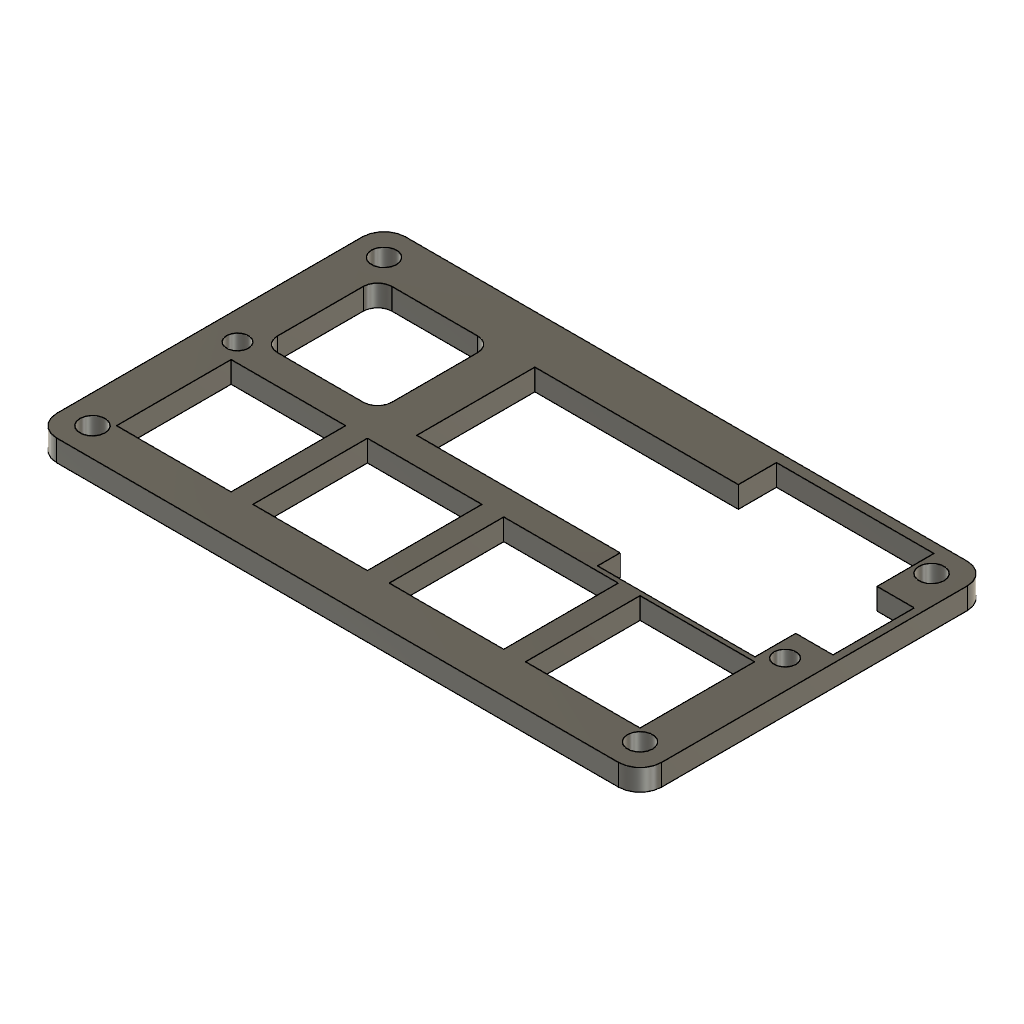
Hayai full bulid V1 (Autodesk Fusion 360 archive; units mm, degrees)
design "Hayai Upper midplate"
part number: 2026-09-20-16-56-58-125
Autodesk Fusion 360 part; units mm, degrees
note: some values were not read from the file. Chosen so that the rebuilt part matches the saved one: which face or edge a step refers to. Set by a fixed rule: which sketch regions a step uses.
(part 1 of 2)
sketch "Sketch1" plane through (0, 0, 0) normal (0, 0, 1) x (1, 0, 0)
  circle A0 centre (-38.26, 20.3675) radius 1.75
  circle A1 centre (38.26, 20.3675) radius 1.75
  circle A2 centre (38.26, -20.3675) radius 1.75
  circle A3 centre (-38.26, -20.3675) radius 1.75
  line L0 (14, 22.9575) -> (36, 22.9575)
  line L1 (36, 15) -> (36, 22.9575)
  line L2 (36, 15) -> (41.21, 15)
  line L3 (41.21, 15) -> (41.21, 3.65)
  line L4 (41.21, 3.65) -> (36, 3.65)
  line L5 (36, -2.0425) -> (36, 3.65)
  line L6 (36, -2.0425) -> (14, -2.0425)
  line L7 (-14.435, 1.1275) -> (-14.435, 17.6275)
  line L8 (-14.435, 1.1275) -> (14, 1.1275)
  line L9 (-14.435, 17.6275) -> (14, 17.6275)
  line L10 (14, -2.0425) -> (14, 1.1275)
  line L11 (14, 17.6275) -> (14, 22.9575)
  circle A4 centre (-38.26, -0.0995) radius 1.525
  circle A5 centre (38.26, -0.0995) radius 1.525
  line L12 (-39.26, 24.3675) -> (39.26, 24.3675)
  line L13 (42.26, 21.3675) -> (42.26, -21.3675)
  line L14 (39.26, -24.3675) -> (-39.26, -24.3675)
  line L15 (-42.26, -21.3675) -> (-42.26, 21.3675)
  arc A6 (-39.26, 24.3675) -> (-42.26, 21.3675) centre (-39.26, 21.3675) ccw
  arc A7 (42.26, 21.3675) -> (39.26, 24.3675) centre (39.26, 21.3675) ccw
  arc A8 (39.26, -24.3675) -> (42.26, -21.3675) centre (39.26, -21.3675) ccw
  arc A9 (-42.26, -21.3675) -> (-39.26, -24.3675) centre (-39.26, -21.3675) ccw
  line L16 (-22.19, 1.4035) -> (-34.19, 1.4035)
  line L17 (-36.19, 3.4035) -> (-36.19, 15.4035)
  line L18 (-34.19, 17.4035) -> (-22.19, 17.4035)
  line L19 (-20.19, 15.4035) -> (-20.19, 3.4035)
  line L20 (-20.19, 1.4035) -> (-36.19, 17.4035) construction
  line L21 (-36.19, 1.4035) -> (-20.19, 17.4035) construction
  arc A10 (-34.19, 17.4035) -> (-36.19, 15.4035) centre (-34.19, 15.4035) ccw
  arc A11 (-22.19, 1.4035) -> (-20.19, 3.4035) centre (-22.19, 3.4035) ccw
  arc A12 (-36.19, 3.4035) -> (-34.19, 1.4035) centre (-34.19, 3.4035) ccw
  arc A13 (-20.19, 15.4035) -> (-22.19, 17.4035) centre (-22.19, 15.4035) ccw
  line L22 (20.575, -18.6825) -> (36.575, -18.6825)
  line L23 (36.575, -18.6825) -> (36.575, -2.6825)
  line L24 (36.575, -2.6825) -> (20.575, -2.6825)
  line L25 (20.575, -2.6825) -> (20.575, -18.6825)
  line L26 (20.575, -18.6825) -> (36.575, -2.6825) construction
  line L27 (36.575, -18.6825) -> (20.575, -2.6825) construction
  line L28 (1.525, -18.6825) -> (17.525, -18.6825)
  line L29 (17.525, -18.6825) -> (17.525, -2.6825)
  line L30 (17.525, -2.6825) -> (1.525, -2.6825)
  line L31 (1.525, -2.6825) -> (1.525, -18.6825)
  line L32 (1.525, -18.6825) -> (17.525, -2.6825) construction
  line L33 (17.525, -18.6825) -> (1.525, -2.6825) construction
  line L34 (-17.525, -18.6825) -> (-1.525, -18.6825)
  line L35 (-1.525, -18.6825) -> (-1.525, -2.6825)
  line L36 (-1.525, -2.6825) -> (-17.525, -2.6825)
  line L37 (-17.525, -2.6825) -> (-17.525, -18.6825)
  line L38 (-17.525, -18.6825) -> (-1.525, -2.6825) construction
  line L39 (-1.525, -18.6825) -> (-17.525, -2.6825) construction
  line L40 (-36.575, -18.6825) -> (-20.575, -18.6825)
  line L41 (-20.575, -18.6825) -> (-20.575, -2.6825)
  line L42 (-20.575, -2.6825) -> (-36.575, -2.6825)
  line L43 (-36.575, -2.6825) -> (-36.575, -18.6825)
  line L44 (-36.575, -18.6825) -> (-20.575, -2.6825) construction
  line L45 (-20.575, -18.6825) -> (-36.575, -2.6825) construction
  point P0 (1.0651, 9.3775)
  point P1 (-28.19, 9.4035)
  point P2 (-28.19, 9.4035)
  point P3 (42.26, -24.3675)
  point P4 (-42.26, 24.3675)
  point P5 (-28.19, 9.4035)
  point P6 (-28.19, 9.4035)
  point P7 (28.575, -10.6825)
  point P8 (9.525, -10.6825)
  point P9 (-28.575, -10.6825)
  point P10 (-9.525, -10.6825)
  point P11 (28.575, -10.6825)
  point P12 (9.525, -10.6825)
  point P13 (-9.525, -10.6825)
  point P14 (-28.575, -10.6825)
  dimension "d2" = 3.5
  dimension "d11" = 22
  dimension "d12" = 25
  dimension "d13" = 5.21
  dimension "d14" = 11.35
  dimension "d18" = 16.5
  dimension "d31" = 3.05
  dimension "d32" = 3.05
  dimension "d33" = 20.268
  dimension "d34" = 20.268
  dimension "d53" = 3
  dimension "d54" = 3
  dimension "d55" = 3
  dimension "d56" = 3
  dimension "d67" = 84.52
  dimension "d68" = 14.07
  dimension "d69" = 14.964
  dimension "d70" = 16
  dimension "d71" = 16
  dimension "d72" = 2
  dimension "d73" = 2
  dimension "d74" = 2
  dimension "d75" = 2
  dimension "d80" = 19.05
  dimension "d81" = 16
  dimension "d82" = 16
  dimension "d83" = 16
  dimension "d84" = 16
  dimension "d85" = 16
  dimension "d86" = 16
  dimension "d87" = 16
  dimension "d88" = 16
  constraint horizontal L0
  constraint horizontal L6
  constraint horizontal L2
  constraint vertical L3
  constraint horizontal L4
  constraint perpendicular L8 L10
  constraint coincident P6 P5
  constraint horizontal L12
  constraint vertical L13
  constraint horizontal L14
  constraint vertical L15
  constraint tangent L12 A6
  constraint tangent L15 A6
  constraint tangent L12 A7
  constraint tangent L13 A7
  constraint tangent L13 A8
  constraint tangent L14 A8
  constraint tangent L14 A9
  constraint tangent L15 A9
  constraint horizontal L16
  constraint perpendicular L16 L17
  constraint parallel L16 L18
  constraint parallel L17 L19
  constraint coincident L20 P6
  constraint coincident L21 P6
  constraint coincident L20.end L18
  constraint coincident L20.end L17
  constraint tangent L18 A10
  constraint tangent L17 A10
  constraint coincident L20.start L16
  constraint coincident L20.start L19
  constraint tangent L16 A11
  constraint tangent L19 A11
  constraint coincident L21.start L16
  constraint coincident L21.start L17
  constraint tangent L16 A12
  constraint tangent L17 A12
  constraint coincident L21.end L18
  constraint coincident L21.end L19
  constraint tangent L18 A13
  constraint tangent L19 A13
  constraint horizontal L22
  constraint perpendicular L22 L23
  constraint parallel L22 L24
  constraint parallel L23 L25
  constraint coincident L26 P11
  constraint coincident L27 P11
  constraint coincident P11 P7
  constraint horizontal L28
  constraint perpendicular L28 L29
  constraint parallel L28 L30
  constraint parallel L29 L31
  constraint coincident L32 P12
  constraint coincident L33 P12
  constraint coincident P12 P8
  constraint horizontal L34
  constraint perpendicular L34 L35
  constraint parallel L34 L36
  constraint parallel L35 L37
  constraint coincident L38 P13
  constraint coincident L39 P13
  constraint coincident P13 P10
  constraint horizontal L40
  constraint perpendicular L40 L41
  constraint parallel L40 L42
  constraint parallel L41 L43
  constraint coincident L44 P14
  constraint coincident L45 P14
  constraint coincident P14 P9
  constraint equal A0 A3
  constraint equal A0 A2
  constraint equal A0 A1
  measures "d2" diameter of A0
  measures "d11" distance of L0.end L0.start
  measures "d12" distance of L6.end L0.start
  measures "d13" distance of L1.start L2.end
  measures "d14" distance of L1.start L4.end
  measures "d18" distance of L7.start L7.end
  measures "d31" diameter of A4
  measures "d32" diameter of A5
  measures "d33" distance of A2.centre A5.centre
  measures "d34" distance of A3.centre A4.centre
  measures "d53" radius of A6
  measures "d54" radius of A7
  measures "d55" radius of A8
  measures "d56" radius of A9
  measures "d67" distance of L13 L15
  measures "d68" distance of L15 P6
  measures "d69" distance of L12 P6
  measures "d70" distance of L20.end L21.end
  measures "d71" distance of L21.start L20.end
  measures "d72" radius of A10
  measures "d73" radius of A11
  measures "d74" radius of A12
  measures "d75" radius of A13
  measures "d80" distance of P14 P13
  measures "d81" distance of L23.end L24.end
  measures "d82" distance of L22.end L23.end
  measures "d83" distance of L29.end L30.end
  measures "d84" distance of L28.end L29.end
  measures "d85" distance of L35.end L36.end
  measures "d86" distance of L34.end L35.end
  measures "d87" distance of L41.end L42.end
  measures "d88" distance of L40.end L41.end
extrude "Extrude13" add sketch "Sketch1" along normal blind 3 contours L12 L13 L14 L15 A6 A7 A8 A9 | L16 L17 L18 L19 A10 A11 A12 A13 | L22 L23 L24 L25 | L28 L29 L30 L31 | L34 L35 L36 L37 | L40 L41 L42 L43 makes body 1
extrude "Extrude14" add sketch "Sketch1" along normal blind 3 separate body contours L12 L13 L14 L15 A6 A7 A8 A9 | L22 L23 L24 L25 | L28 L29 L30 L31 | L34 L35 L36 L37 | L40 L41 L42 L43 makes body 2
extrude "Extrude15" cut sketch "Sketch1" along normal blind 3 contours L16 L17 L18 L19 A10 A11 A12 A13 bodies 1
extrude "Extrude16" add sketch "Sketch1" along normal blind 3 separate body makes body 3
extrude "Extrude17" cut sketch "Sketch1" along normal blind 3 contours L22 L23 L24 L25 | L28 L29 L30 L31 | L34 L35 L36 L37 | L40 L41 L42 L43 bodies 1 2
extrude "Extrude18" add sketch "Sketch1" along normal blind 3 separate body makes body 4

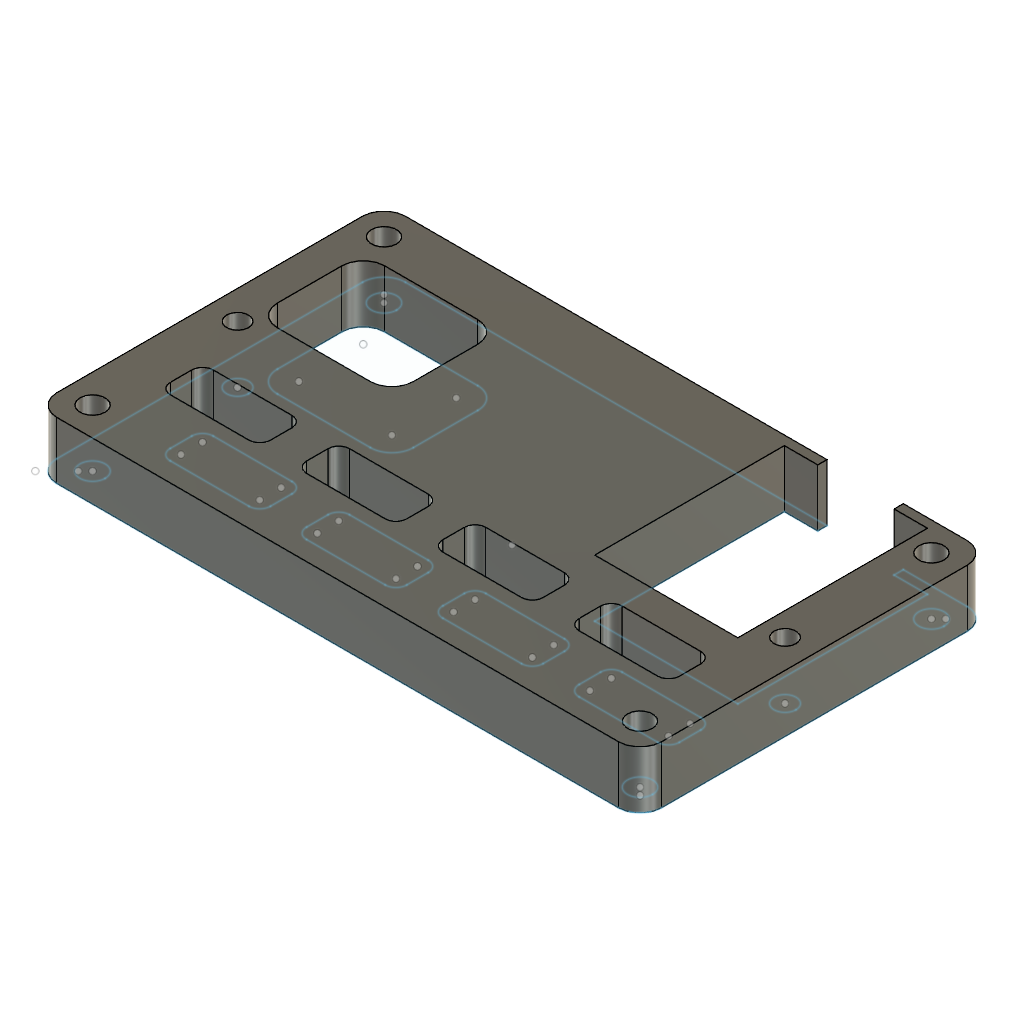
design "Hayai Lower midplate"
part number: 2026-09-20-19-27-11-121
Autodesk Fusion 360 part; units mm, degrees
sketch "Sketch1" plane through (0, 0, 0) normal (0, 0, 1) x (1, 0, 0)
  arc A0 (39.26, -24.3675) -> (42.26, -21.3675) centre (39.26, -21.3675) ccw
  circle A1 centre (38.26, -0.0995) radius 1.525
  circle A2 centre (-38.26, -20.3675) radius 1.75
  circle A3 centre (-38.26, 20.3675) radius 1.75
  line L0 (42.26, 21.3675) -> (42.26, -21.3675)
  arc A4 (-42.26, -21.3675) -> (-39.26, -24.3675) centre (-39.26, -21.3675) ccw
  line L1 (39.26, -24.3675) -> (-39.26, -24.3675)
  line L2 (-42.26, -21.3675) -> (-42.26, 21.3675)
  arc A5 (-39.26, 24.3675) -> (-42.26, 21.3675) centre (-39.26, 21.3675) ccw
  arc A6 (42.26, 21.3675) -> (39.26, 24.3675) centre (39.26, 21.3675) ccw
  circle A7 centre (38.26, 20.3675) radius 1.75
  circle A8 centre (-38.26, -0.0995) radius 1.525
  circle A9 centre (38.26, -20.3675) radius 1.75
  arc A10 (16.525, -9.1875) -> (15.025, -7.6875) centre (15.025, -9.1875) ccw
  arc A11 (-35.575, -12.1875) -> (-34.075, -13.6875) centre (-34.075, -12.1875) ccw
  line L3 (4.025, -7.6875) -> (15.025, -7.6875)
  arc A12 (-15.025, -7.6875) -> (-16.525, -9.1875) centre (-15.025, -9.1875) ccw
  line L4 (-16.525, -12.1875) -> (-16.525, -9.1875)
  line L5 (23.075, -13.6875) -> (34.075, -13.6875)
  line L6 (-15.025, -13.6875) -> (-4.025, -13.6875)
  arc A13 (21.575, -12.1875) -> (23.075, -13.6875) centre (23.075, -12.1875) ccw
  line L7 (-34.075, -7.6875) -> (-23.075, -7.6875)
  arc A14 (34.075, -13.6875) -> (35.575, -12.1875) centre (34.075, -12.1875) ccw
  line L8 (-34.075, -13.6875) -> (-23.075, -13.6875)
  line L9 (2.525, -12.1875) -> (2.525, -9.1875)
  arc A15 (35.575, -9.1875) -> (34.075, -7.6875) centre (34.075, -9.1875) ccw
  arc A16 (-2.525, -9.1875) -> (-4.025, -7.6875) centre (-4.025, -9.1875) ccw
  arc A17 (4.025, -7.6875) -> (2.525, -9.1875) centre (4.025, -9.1875) ccw
  line L10 (-35.575, -12.1875) -> (-35.575, -9.1875)
  line L11 (16.525, -12.1875) -> (16.525, -9.1875)
  arc A18 (-4.025, -13.6875) -> (-2.525, -12.1875) centre (-4.025, -12.1875) ccw
  line L12 (23.075, -7.6875) -> (34.075, -7.6875)
  arc A19 (-23.075, -13.6875) -> (-21.575, -12.1875) centre (-23.075, -12.1875) ccw
  line L13 (21.575, -12.1875) -> (21.575, -9.1875)
  line L14 (-15.025, -7.6875) -> (-4.025, -7.6875)
  line L15 (35.575, -12.1875) -> (35.575, -9.1875)
  arc A20 (2.525, -12.1875) -> (4.025, -13.6875) centre (4.025, -12.1875) ccw
  arc A21 (-16.525, -12.1875) -> (-15.025, -13.6875) centre (-15.025, -12.1875) ccw
  arc A22 (-21.575, -9.1875) -> (-23.075, -7.6875) centre (-23.075, -9.1875) ccw
  line L16 (-21.575, -12.1875) -> (-21.575, -9.1875)
  line L17 (-2.525, -12.1875) -> (-2.525, -9.1875)
  arc A23 (15.025, -13.6875) -> (16.525, -12.1875) centre (15.025, -12.1875) ccw
  arc A24 (-34.075, -7.6875) -> (-35.575, -9.1875) centre (-34.075, -9.1875) ccw
  line L18 (4.025, -13.6875) -> (15.025, -13.6875)
  arc A25 (23.075, -7.6875) -> (21.575, -9.1875) centre (23.075, -9.1875) ccw
  line L19 (-18.69, 4.8975) -> (-18.69, 13.8975)
  arc A26 (-18.69, 13.8975) -> (-21.69, 16.8975) centre (-21.69, 13.8975) ccw
  line L20 (-21.69, 16.8975) -> (-34.69, 16.8975)
  arc A27 (-34.69, 16.8975) -> (-37.69, 13.8975) centre (-34.69, 13.8975) ccw
  line L21 (-37.69, 4.8975) -> (-37.69, 13.8975)
  arc A28 (-37.69, 4.8975) -> (-34.69, 1.8975) centre (-34.69, 4.8975) ccw
  line L22 (-21.69, 1.8975) -> (-34.69, 1.8975)
  arc A29 (-21.69, 1.8975) -> (-18.69, 4.8975) centre (-21.69, 4.8975) ccw
  line L23 (35, -3.4325) -> (15, -3.4325)
  line L24 (19.67, 23.0675) -> (15, 23.0675)
  line L25 (30.33, 23.0675) -> (35, 23.0675)
  line L26 (15, -3.4325) -> (15, 23.0675)
  line L27 (35, 23.0675) -> (35, -3.4325)
  line L28 (19.67, 23.0675) -> (19.67, 24.3675)
  line L29 (30.33, 23.0675) -> (30.33, 24.3675)
  line L30 (39.26, 24.3675) -> (30.33, 24.3675)
  line L31 (19.67, 24.3675) -> (-39.26, 24.3675)
  point P0 (-42.26, -24.3675)
  dimension "d1" = 3.5
  dimension "d2" = 3.05
  dimension "d3" = 3.05
  dimension "d4" = 20.268
  dimension "d5" = 3
  dimension "d6" = 3
  dimension "d7" = 3
  dimension "d8" = 3
  dimension "d11" = 3.5
  dimension "d12" = 1.4142
  dimension "d13" = 4
  dimension "d14" = 10.68
  dimension "d15" = 6
  dimension "d16" = 14
  dimension "d17" = 1.5
  dimension "d18" = 1.5
  dimension "d19" = 1.5
  dimension "d20" = 1.5
  dimension "d21" = 1.5
  dimension "d22" = 1.5
  dimension "d23" = 1.5
  dimension "d24" = 1.5
  dimension "d25" = 1.5
  dimension "d26" = 1.5
  dimension "d27" = 1.5
  dimension "d28" = 1.5
  dimension "d29" = 1.5
  dimension "d30" = 1.5
  dimension "d31" = 1.5
  dimension "d32" = 1.5
  dimension "d33" = 6
  dimension "d34" = 6
  dimension "d35" = 6
  dimension "d36" = 10.68
  dimension "d37" = 10.68
  dimension "d38" = 10.68
  dimension "d40" = 6.685
  dimension "d41" = 5.05
  dimension "d42" = 5.05
  dimension "d43" = 5.05
  dimension "d44" = 4
  dimension "d45" = 4
  dimension "d46" = 4
  dimension "d47" = 1.4142
  dimension "d48" = 4
  dimension "d49" = 1.4142
  dimension "d50" = 20.268
  dimension "d51" = 14
  dimension "d52" = 14
  dimension "d53" = 14
  dimension "d54" = 6.685
  dimension "d55" = 3
  dimension "d56" = 3
  dimension "d57" = 3
  dimension "d58" = 3
  dimension "d59" = 19
  dimension "d60" = 15
  dimension "d61" = 4.57
  dimension "d63" = 26.5
  dimension "d64" = 26.5
  dimension "d65" = 20
  dimension "d66" = 10.66
  dimension "d67" = 1.3
  dimension "d68" = 1.3
  dimension "d69" = 4.67
  dimension "d70" = 4.67
  dimension "d71" = 7.26
  dimension "d78" = 3.5
  dimension "d79" = 3.5
  constraint vertical L0
  constraint horizontal L1
  constraint vertical L2
  constraint tangent L2 A5
  constraint tangent L0 A6
  constraint tangent A0 L0
  constraint tangent A0 L1
  constraint tangent A4 L1
  constraint tangent A4 L2
  constraint tangent A6 L30
  constraint tangent A5 L31
  measures "d1" diameter of A3
  measures "d2" diameter of A8
  measures "d3" diameter of A1
  measures "d4" distance of A2.centre A8.centre
  measures "d5" radius of A5
  measures "d6" radius of A6
  measures "d7" radius of A0
  measures "d8" radius of A4
  measures "d11" diameter of A9
  measures "d12" distance of A0.centre A9.centre
  measures "d13" distance of L1 A9.centre
  measures "d14" distance of L1 L8
  measures "d15" distance of L7 L8
  measures "d16" distance of L10 L16
  measures "d17" radius of A19
  measures "d18" radius of A22
  measures "d19" radius of A24
  measures "d20" radius of A11
  measures "d21" radius of A21
  measures "d22" radius of A12
  measures "d23" radius of A16
  measures "d24" radius of A18
  measures "d25" radius of A20
  measures "d26" radius of A17
  measures "d27" radius of A10
  measures "d28" radius of A23
  measures "d29" radius of A13
  measures "d30" radius of A25
  measures "d31" radius of A15
  measures "d32" radius of A14
  measures "d33" distance of L6 L14
  measures "d34" distance of L3 L18
  measures "d35" distance of L5 L12
  measures "d36" distance of L1 L6
  measures "d37" distance of L1 L5
  measures "d38" distance of L1 L18
  measures "d40" distance of L2 L10
  measures "d41" distance of L4 L16
  measures "d42" distance of L9 L17
  measures "d43" distance of L11 L13
  measures "d44" distance of A8.centre L2
  measures "d45" distance of A3.centre L2
  measures "d46" distance of A7.centre L0
  measures "d47" distance of A6.centre A7.centre
  measures "d48" distance of A1.centre L0
  measures "d49" distance of A5.centre A3.centre
  measures "d50" distance of A1.centre A9.centre
  measures "d51" distance of L4 L17
  measures "d52" distance of L9 L11
  measures "d53" distance of L13 L15
  measures "d54" distance of L0 L15
  measures "d55" radius of A28
  measures "d56" radius of A29
  measures "d57" radius of A26
  measures "d58" radius of A27
  measures "d59" distance of L19 L21
  measures "d60" distance of L20 L22
  measures "d61" distance of L2 L21
  measures "d63" distance of L23 L24
  measures "d64" distance of L23 L25
  measures "d65" distance of L26 L27
  measures "d66" distance of L28 L29
  measures "d67" distance of L24.start L28.end
  measures "d68" distance of L29.end L25.start
  measures "d69" distance of L24.end L28
  measures "d70" distance of L25.end L29
  measures "d71" distance of L0 L27
  measures "d78" diameter of A2
  measures "d79" diameter of A7
extrude "Extrude1" add sketch "Sketch1" along normal blind 3
extrude "Extrude2" add 1 faces at (0.0405, 9.7541, 3) along direction (0, 0, 1) blind 4
extrude "Extrude4" add 1 faces at (0.0405, 9.7541, 7) along direction (0, 0, 1) blind 1

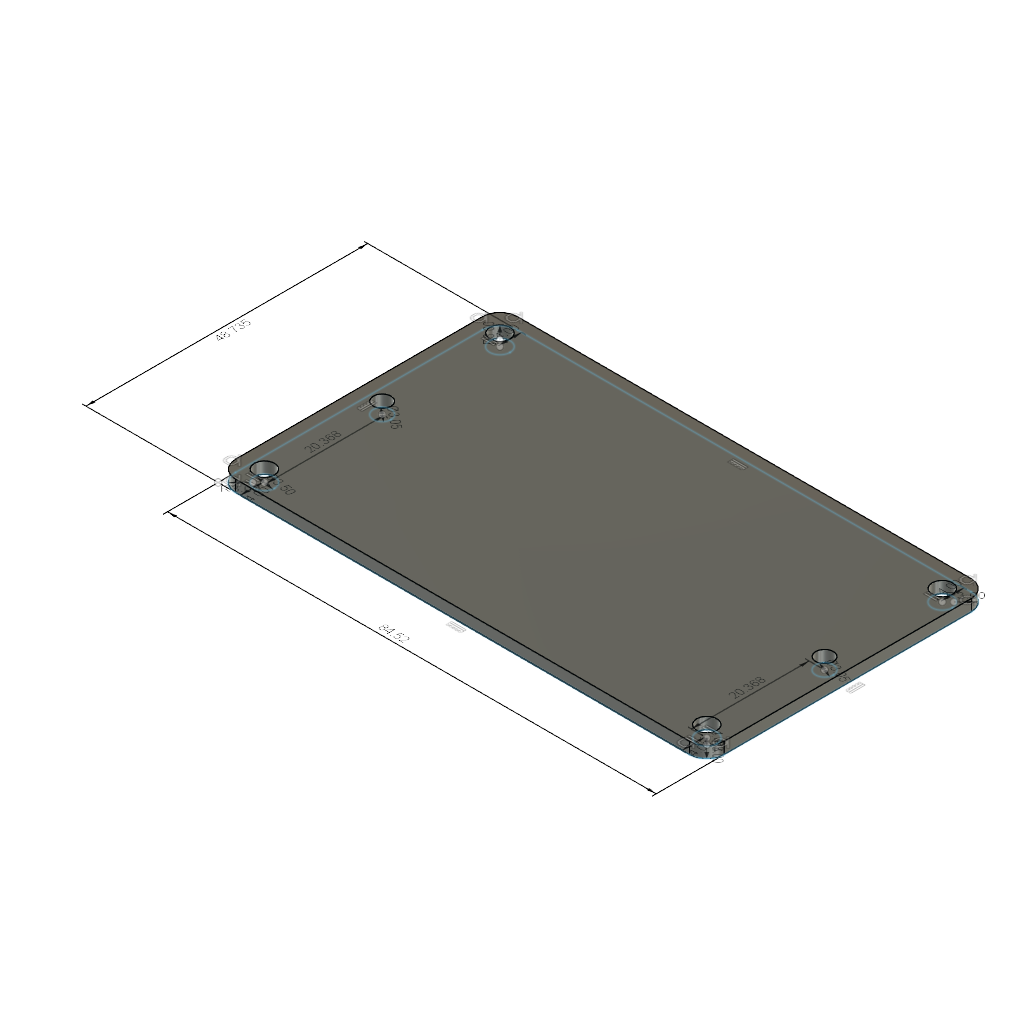
design "Hayai Bottom plate"
part number: 2026-09-20-15-42-52-633
Autodesk Fusion 360 part; units mm, degrees
sketch "Sketch1" plane through (0, 0, 0) normal (0, 0, 1) x (1, 0, 0)
  circle A0 centre (38.26, 20.3675) radius 1.75
  circle A1 centre (38.26, 0.0005) radius 1.525
  circle A2 centre (-38.26, -20.3675) radius 1.75
  circle A3 centre (-38.26, 20.3675) radius 1.75
  arc A4 (-39.26, 24.3675) -> (-42.26, 21.3675) centre (-39.26, 21.3675) ccw
  line L0 (-39.26, 24.3675) -> (39.26, 24.3675)
  line L1 (-42.26, -21.3675) -> (-42.26, 21.3675)
  circle A5 centre (-38.26, 0.0005) radius 1.525
  arc A6 (42.26, 21.3675) -> (39.26, 24.3675) centre (39.26, 21.3675) ccw
  line L2 (42.26, 21.3675) -> (42.26, -21.3675)
  arc A7 (-42.26, -21.3675) -> (-39.26, -24.3675) centre (-39.26, -21.3675) ccw
  line L3 (39.26, -24.3675) -> (-39.26, -24.3675)
  arc A8 (39.26, -24.3675) -> (42.26, -21.3675) centre (39.26, -21.3675) ccw
  circle A9 centre (38.26, -20.3675) radius 1.75
  point P0 (-42.26, -24.3675)
  dimension "d32" = 3.05
  dimension "d33" = 3.05
  dimension "d34" = 20.368
  dimension "d35" = 3
  dimension "d36" = 3
  dimension "d37" = 3
  dimension "d38" = 3
  dimension "d41" = 1.4142
  dimension "d42" = 4
  dimension "d45" = 4
  dimension "d51" = 20.368
  dimension "d52" = 48.735
  dimension "d55" = 4
  dimension "d56" = 4
  dimension "d59" = 3.5
  dimension "d62" = 84.52
  constraint horizontal L0
  constraint vertical L2
  constraint horizontal L3
  constraint vertical L1
  constraint tangent A4 L0
  constraint tangent A4 L1
  constraint tangent L0 A6
  constraint tangent A6 L2
  constraint tangent L2 A8
  constraint tangent L3 A8
  constraint tangent A7 L3
  constraint tangent L1 A7
  constraint equal A2 A3
  constraint equal A0 A9
  constraint equal A2 A9
  measures "d32" diameter of A5
  measures "d33" diameter of A1
  measures "d34" distance of A5.centre A2.centre
  measures "d35" radius of A4
  measures "d36" radius of A6
  measures "d37" radius of A8
  measures "d38" radius of A7
  measures "d41" distance of A8.centre A9.centre
  measures "d42" distance of L3 A9.centre
  measures "d45" distance of A3.centre L0
  measures "d51" distance of A1.centre A9.centre
  measures "d52" distance of L0 L3
  measures "d55" distance of A2.centre L3
  measures "d56" distance of A0.centre L0
  measures "d59" diameter of A2
  measures "d62" distance of L1 L2
extrude "Extrude1" add sketch "Sketch1" along normal blind 2 contours A4 L0 L1 A6 L2 A7 L3 A8 | A9 makes body 1
extrude "Extrude2" add sketch "Sketch1" along normal blind 2 separate body contours A4 L0 L1 A6 L2 A7 L3 A8 | A9 makes body 2
extrude "Extrude3" add sketch "Sketch1" along normal blind 2 separate body makes body 3
extrude "Extrude4" cut sketch "Sketch1" along normal blind 2 contours A9 bodies 1 2
extrude "Extrude5" add sketch "Sketch1" along normal blind 2 separate body makes body 4
extrude "Extrude6" add sketch "Sketch1" along normal blind 2 separate body makes body 5
extrude "Extrude7" add sketch "Sketch1" along normal blind 2 separate body makes body 6
equation "d41 = ( sqrt(2) ) * 1 mm"

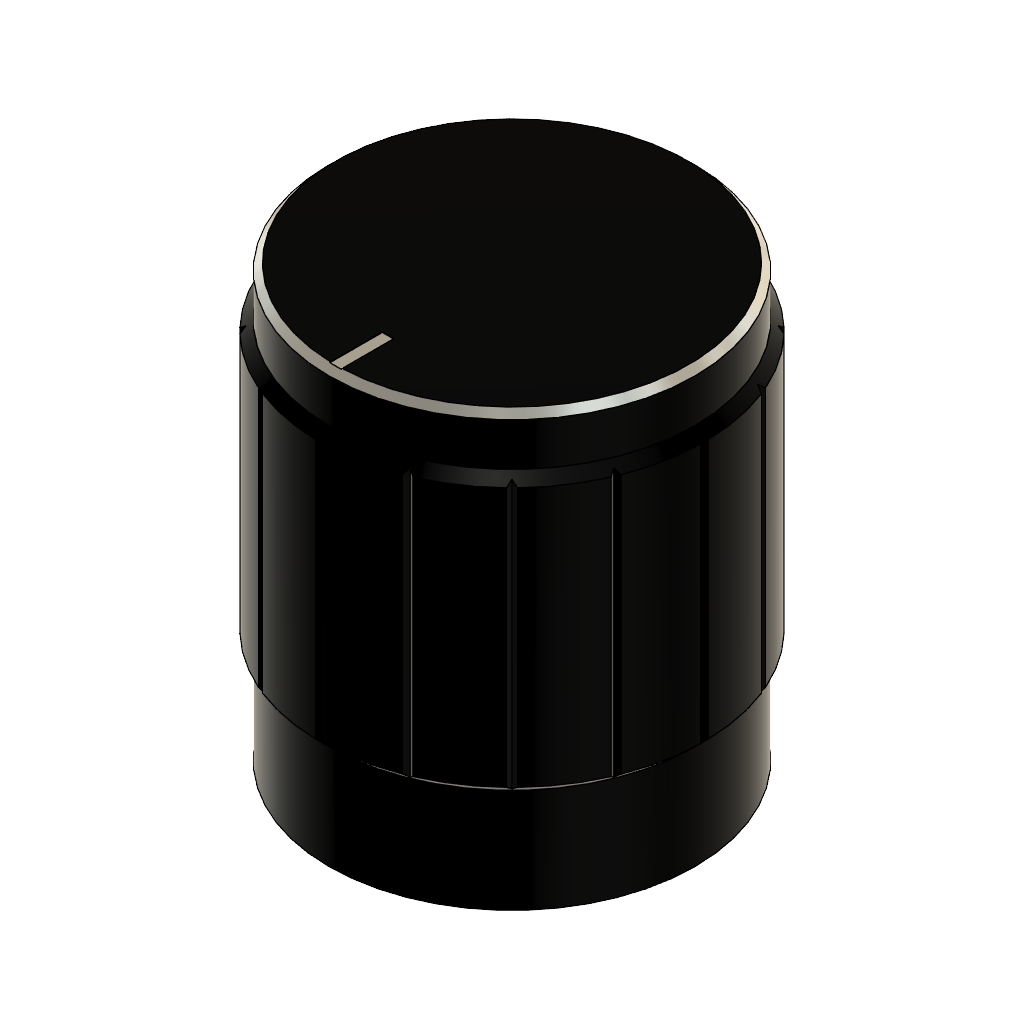
design "encoder cap"
Autodesk Fusion 360 part; units mm, degrees
sketch "Board" plane through (0, 0, 0) normal (0, 0, 1) x (1, 0, 0)
  line L0 (9.5, -13.125) -> (-9.5, -13.125)
  line L1 (-9.5, -13.125) -> (-9.5, 13.125)
  line L2 (-9.5, 13.125) -> (9.5, 13.125)
  line L3 (9.5, 13.125) -> (9.5, -13.125)
  line L4 (9.5, -13.125) -> (-9.5, 13.125) construction
  line L5 (-9.5, -13.125) -> (9.5, 13.125) construction
  line L6 (-9.5, 8.775) -> (9.5, 8.775) construction
  line L7 (-7, -13.125) -> (-7, 13.125) construction
  circle A0 centre (-7, 8.775) radius 1.5
  line L8 (-7, 8.775) -> (-7, -8.075) construction
  circle A1 centre (-7, -8.075) radius 1.5
  line L9 (9.5, -9.125) -> (-9.5, -9.125) construction
  line L10 (9.5, -11.575) -> (-9.5, -11.575) construction
  line L11 (8.3, 13.125) -> (8.3, -13.125) construction
  line L12 (-4.25, 13.125) -> (-4.25, -13.125) construction
  line L13 (-4.25, -9.125) -> (-1.74, -9.125)
  line L14 (-1.74, -9.125) -> (-1.74, -11.575)
  line L15 (-1.74, -11.575) -> (-4.25, -11.575)
  line L16 (-4.25, -11.575) -> (-4.25, -9.125)
  line L17 (-1.74, -9.125) -> (0.77, -9.125)
  line L18 (0.77, -9.125) -> (0.77, -11.575)
  line L19 (0.77, -11.575) -> (-1.74, -11.575)
  line L20 (-1.74, -11.575) -> (-1.74, -9.125)
  line L21 (0.77, -9.125) -> (3.28, -9.125)
  line L22 (3.28, -9.125) -> (3.28, -11.575)
  line L23 (3.28, -11.575) -> (0.77, -11.575)
  line L24 (0.77, -11.575) -> (0.77, -9.125)
  line L25 (3.28, -9.125) -> (5.79, -9.125)
  line L26 (5.79, -9.125) -> (5.79, -11.575)
  line L27 (5.79, -11.575) -> (3.28, -11.575)
  line L28 (3.28, -11.575) -> (3.28, -9.125)
  line L29 (5.79, -9.125) -> (8.3, -9.125)
  line L30 (8.3, -9.125) -> (8.3, -11.575)
  line L31 (8.3, -11.575) -> (5.79, -11.575)
  line L32 (5.79, -11.575) -> (5.79, -9.125)
  line L33 (-4.25, -10.35) -> (-1.74, -10.35) construction
  line L34 (-1.74, -10.35) -> (0.77, -10.35) construction
  line L35 (0.77, -10.35) -> (3.28, -10.35) construction
  line L36 (3.28, -10.35) -> (5.79, -10.35) construction
  line L37 (5.79, -10.35) -> (8.3, -10.35) construction
  circle A2 centre (-2.995, -10.35) radius 0.5
  circle A3 centre (-0.485, -10.35) radius 0.5
  circle A4 centre (2.025, -10.35) radius 0.5
  circle A5 centre (4.535, -10.35) radius 0.5
  circle A6 centre (7.045, -10.35) radius 0.5
  dimension "d1" = 19
  dimension "d2" = 26.25
  dimension "d3" = 4.35
  dimension "d4" = 2.5
  dimension "d5" = 3
  dimension "d6" = 16.85
  dimension "d7" = 3
  dimension "d8" = 4
  dimension "d9" = 1.55
  dimension "d10" = 1.2
  dimension "d11" = 13.75
  dimension "d12" = 2.51
  dimension "d13" = 2.51
  dimension "d14" = 2.51
  dimension "d15" = 2.51
  dimension "d16" = 2.51
  dimension "d17" = 1
  dimension "d18" = 1
  dimension "d19" = 1
  dimension "d20" = 1
  dimension "d21" = 1
  constraint horizontal L0
  constraint perpendicular L0 L1
  constraint parallel L0 L2
  constraint parallel L1 L3
  constraint coincident L4 origin
  constraint coincident L5 origin
  constraint coincident L6 A0.centre
  constraint coincident L7 A0.centre
  constraint coincident A0.centre L8.start
  constraint perpendicular L6 L8
  constraint coincident L8.end A1.centre
  constraint horizontal L13
  constraint vertical L14
  constraint horizontal L15
  constraint vertical L16
  constraint coincident L12 L13.start
  constraint coincident L9 L13.start
  constraint horizontal L17
  constraint vertical L18
  constraint horizontal L19
  constraint vertical L20
  constraint horizontal L21
  constraint vertical L22
  constraint horizontal L23
  constraint vertical L24
  constraint horizontal L25
  constraint vertical L26
  constraint horizontal L27
  constraint vertical L28
  constraint horizontal L29
  constraint vertical L30
  constraint horizontal L31
  constraint vertical L32
  constraint midpoint L16 L33.start
  constraint midpoint L20 L33.end
  constraint perpendicular L20 L33
  constraint midpoint L24 L34.end
  constraint perpendicular L24 L34
  constraint midpoint L28 L35.end
  constraint perpendicular L28 L35
  constraint midpoint L32 L36.end
  constraint perpendicular L32 L36
  constraint midpoint L30 L37.end
  constraint midpoint L33 A2.centre
  constraint midpoint L34 A3.centre
  constraint midpoint L35 A4.centre
  constraint midpoint L36 A5.centre
  constraint midpoint L37 A6.centre
  measures "d1" distance of L1.end L2.end
  measures "d2" distance of L0.end L1.end
  measures "d5" diameter of A0
  measures "d6" distance of A0.centre L8.end
  measures "d7" diameter of A1
  measures "d12" distance of L13.start L13.end
  measures "d13" distance of L13.end L17.end
  measures "d14" distance of L17.end L21.end
  measures "d15" distance of L21.end L25.end
  measures "d16" distance of L25.end L29.end
  measures "d17" diameter of A2
  measures "d18" diameter of A3
  measures "d19" diameter of A4
  measures "d20" diameter of A5
  measures "d21" diameter of A6
sketch "Encoder I" plane through (0, 0, 0) normal (0, 0, 1) x (1, 0, 0)
  line L0 (9.5, 13.125) -> (9.5, -13.125) construction
  line L1 (-9.5, 13.125) -> (9.5, 13.125) construction
  line L2 (7.5, 13.125) -> (7.5, -13.125) construction
  line L3 (-9.5, 8.465) -> (9.5, 8.465) construction
  line L4 (7.5, 8.465) -> (-4.4, 8.465)
  line L5 (-4.4, 8.465) -> (-4.4, -3.435)
  line L6 (-4.4, -3.435) -> (7.5, -3.435)
  line L7 (7.5, -3.435) -> (7.5, 8.465)
  line L8 (1.55, 8.465) -> (1.55, -3.435) construction
  line L9 (-1.68, 2.515) -> (4.78, 2.515) construction
  line L10 (4.78, 2.515) -> (4.78, 8.465) construction
  line L11 (-1.68, 2.515) -> (-1.68, 8.465) construction
  line L12 (4.78, 2.515) -> (4.78, -3.435) construction
  line L13 (-1.68, 2.515) -> (-1.68, -3.435) construction
  line L14 (4.78, 8.465) -> (4.78, 10.115) construction
  line L15 (1.55, 8.465) -> (1.55, 10.115) construction
  line L16 (-1.68, 8.465) -> (-1.68, 10.115) construction
  line L17 (4.78, -3.435) -> (4.78, -4.535) construction
  line L18 (-1.68, -3.435) -> (-1.68, -4.535) construction
  line L19 (5.53, 8.465) -> (4.03, 8.465)
  line L20 (4.03, 8.465) -> (4.03, 10.115)
  line L21 (4.03, 10.115) -> (5.53, 10.115)
  line L22 (5.53, 10.115) -> (5.53, 8.465)
  line L23 (5.53, 8.465) -> (4.03, 10.115) construction
  line L24 (4.03, 8.465) -> (5.53, 10.115) construction
  line L25 (2.3, 8.465) -> (0.8, 8.465)
  line L26 (0.8, 8.465) -> (0.8, 10.115)
  line L27 (0.8, 10.115) -> (2.3, 10.115)
  line L28 (2.3, 10.115) -> (2.3, 8.465)
  line L29 (2.3, 8.465) -> (0.8, 10.115) construction
  line L30 (0.8, 8.465) -> (2.3, 10.115) construction
  line L31 (-0.93, 8.465) -> (-2.43, 8.465)
  line L32 (-2.43, 8.465) -> (-2.43, 10.115)
  line L33 (-2.43, 10.115) -> (-0.93, 10.115)
  line L34 (-0.93, 10.115) -> (-0.93, 8.465)
  line L35 (-0.93, 8.465) -> (-2.43, 10.115) construction
  line L36 (-2.43, 8.465) -> (-0.93, 10.115) construction
  line L37 (5.53, -3.435) -> (4.03, -3.435)
  line L38 (4.03, -3.435) -> (4.03, -4.535)
  line L39 (4.03, -4.535) -> (5.53, -4.535)
  line L40 (5.53, -4.535) -> (5.53, -3.435)
  line L41 (5.53, -3.435) -> (4.03, -4.535) construction
  line L42 (4.03, -3.435) -> (5.53, -4.535) construction
  line L43 (-0.93, -3.435) -> (-2.43, -3.435)
  line L44 (-2.43, -3.435) -> (-2.43, -4.535)
  line L45 (-2.43, -4.535) -> (-0.93, -4.535)
  line L46 (-0.93, -4.535) -> (-0.93, -3.435)
  line L47 (-0.93, -3.435) -> (-2.43, -4.535) construction
  line L48 (-2.43, -3.435) -> (-0.93, -4.535) construction
  circle A0 centre (4.78, 10.115) radius 0.5
  circle A1 centre (1.55, 10.115) radius 0.5
  circle A2 centre (-1.68, 10.115) radius 0.5
  circle A3 centre (-1.68, -4.535) radius 0.5
  circle A4 centre (4.78, -4.535) radius 0.5
  point P0 (4.78, 9.29)
  point P1 (1.55, 9.29)
  point P2 (-1.68, 9.29)
  point P3 (4.78, -3.985)
  point P4 (-1.68, -3.985)
  dimension "d30" = 2
  dimension "d31" = 4.66
  dimension "d32" = 11.9
  dimension "d33" = 11.9
  dimension "d34" = 6.46
  dimension "d35" = 1.65
  dimension "d36" = 1.65
  dimension "d37" = 1.65
  dimension "d38" = 1.1
  dimension "d39" = 1.1
  dimension "d40" = 1.5
  dimension "d41" = 1.5
  dimension "d42" = 1.5
  dimension "d43" = 1.5
  dimension "d44" = 1.5
  dimension "d45" = 1
  dimension "d46" = 1
  dimension "d47" = 1
  dimension "d48" = 1
  dimension "d49" = 1
  constraint horizontal L4
  constraint vertical L5
  constraint horizontal L6
  constraint vertical L7
  constraint coincident L3 L4.start
  constraint coincident L2 L4.start
  constraint midpoint L4 L8.start
  constraint midpoint L6 L8.end
  constraint horizontal L9
  constraint midpoint L8 L9
  constraint vertical L10
  constraint coincident L4 L10.end
  constraint vertical L11
  constraint coincident L4 L11.end
  constraint coincident L6 L12.end
  constraint perpendicular L6 L12
  constraint coincident L6 L13.end
  constraint perpendicular L6 L13
  constraint perpendicular L4 L14
  constraint perpendicular L4 L15
  constraint perpendicular L3 L16
  constraint perpendicular L6 L17
  constraint perpendicular L6 L18
  constraint horizontal L19
  constraint perpendicular L19 L20
  constraint parallel L19 L21
  constraint parallel L20 L22
  constraint coincident L23 P0
  constraint coincident L24 P0
  constraint midpoint L14 P0
  constraint horizontal L25
  constraint perpendicular L25 L26
  constraint parallel L25 L27
  constraint parallel L26 L28
  constraint coincident L29 P1
  constraint coincident L30 P1
  constraint midpoint L15 P1
  constraint horizontal L31
  constraint perpendicular L31 L32
  constraint parallel L31 L33
  constraint parallel L32 L34
  constraint coincident L35 P2
  constraint coincident L36 P2
  constraint midpoint L16 P2
  constraint horizontal L37
  constraint perpendicular L37 L38
  constraint parallel L37 L39
  constraint parallel L38 L40
  constraint coincident L41 P3
  constraint coincident L42 P3
  constraint midpoint L17 P3
  constraint horizontal L43
  constraint perpendicular L43 L44
  constraint parallel L43 L45
  constraint parallel L44 L46
  constraint coincident L47 P4
  constraint coincident L48 P4
  constraint midpoint L18 P4
  constraint coincident L14.end A0.centre
  constraint coincident L15.end A1.centre
  constraint coincident L16.end A2.centre
  constraint coincident L18.end A3.centre
  constraint coincident L17.end A4.centre
  measures "d32" distance of L4.start L4.end
  measures "d33" distance of L4.start L6.end
  measures "d34" distance of L9.start L9.end
  measures "d35" distance of L10.end L14.end
  measures "d36" distance of L8.start L15.end
  measures "d37" distance of L11.end L16.end
  measures "d38" distance of L12.end L17.end
  measures "d39" distance of L13.end L18.end
  measures "d40" distance of L20.end L21.end
  measures "d41" distance of L26.end L27.end
  measures "d42" distance of L32.end L33.end
  measures "d43" distance of L38.end L39.end
  measures "d44" distance of L44.end L45.end
  measures "d45" diameter of A0
  measures "d46" diameter of A1
  measures "d47" diameter of A2
  measures "d48" diameter of A3
  measures "d49" diameter of A4
sketch "Encoder Contact Profiles" plane through (5.53, 0, 0) normal (1, 0, 0) x (0, 1, 0)
  line L0 (8.465, 0) -> (10.115, 0)
  line L1 (10.115, 0) -> (10.115, 1.5)
  line L2 (10.115, 1.5) -> (8.465, 1.5)
  line L3 (8.465, 1.5) -> (8.465, 0)
  line L4 (-4.535, 0) -> (-3.435, 0)
  line L5 (-3.435, 0) -> (-3.435, 1.5)
  line L6 (-3.435, 1.5) -> (-4.535, 1.5)
  line L7 (-4.535, 1.5) -> (-4.535, 0)
  line L8 (10.115, 1.35) -> (8.465, 1.35)
  line L9 (9.965, 0) -> (9.965, 1.5)
  line L10 (-4.385, 1.5) -> (-4.385, 0)
  line L11 (-3.435, 1.35) -> (-4.535, 1.35)
  dimension "d62" = -0.15
  dimension "d63" = -0.15
  dimension "d64" = -0.15
  dimension "d65" = -0.15
sketch "PCB Contacts" plane through (0, 0, 2.6) normal (0, 0, 1) x (-1, 0, 0)
  line L0 (4.25, 10.35) -> (1.74, 10.35) construction
  line L1 (1.74, 10.35) -> (-0.77, 10.35) construction
  line L2 (-0.77, 10.35) -> (-3.28, 10.35) construction
  line L3 (-3.28, 10.35) -> (-5.79, 10.35) construction
  line L4 (-5.79, 10.35) -> (-8.3, 10.35) construction
  line L5 (2.67, 10.675) -> (3.32, 10.675) construction
  line L6 (3.32, 10.675) -> (3.32, 10.025) construction
  line L7 (3.32, 10.025) -> (2.67, 10.025) construction
  line L8 (2.67, 10.025) -> (2.67, 10.675) construction
  line L9 (2.67, 10.675) -> (3.32, 10.025) construction
  line L10 (3.32, 10.675) -> (2.67, 10.025) construction
  line L11 (0.16, 10.675) -> (0.81, 10.675) construction
  line L12 (0.81, 10.675) -> (0.81, 10.025) construction
  line L13 (0.81, 10.025) -> (0.16, 10.025) construction
  line L14 (0.16, 10.025) -> (0.16, 10.675) construction
  line L15 (0.16, 10.675) -> (0.81, 10.025) construction
  line L16 (0.81, 10.675) -> (0.16, 10.025) construction
  line L17 (-2.35, 10.675) -> (-1.7, 10.675) construction
  line L18 (-1.7, 10.675) -> (-1.7, 10.025) construction
  line L19 (-1.7, 10.025) -> (-2.35, 10.025) construction
  line L20 (-2.35, 10.025) -> (-2.35, 10.675) construction
  line L21 (-2.35, 10.675) -> (-1.7, 10.025) construction
  line L22 (-1.7, 10.675) -> (-2.35, 10.025) construction
  line L23 (-4.86, 10.675) -> (-4.21, 10.675) construction
  line L24 (-4.21, 10.675) -> (-4.21, 10.025) construction
  line L25 (-4.21, 10.025) -> (-4.86, 10.025) construction
  line L26 (-4.86, 10.025) -> (-4.86, 10.675) construction
  line L27 (-4.86, 10.675) -> (-4.21, 10.025) construction
  line L28 (-4.21, 10.675) -> (-4.86, 10.025) construction
  line L29 (-7.37, 10.675) -> (-6.72, 10.675) construction
  line L30 (-6.72, 10.675) -> (-6.72, 10.025) construction
  line L31 (-6.72, 10.025) -> (-7.37, 10.025) construction
  line L32 (-7.37, 10.025) -> (-7.37, 10.675) construction
  line L33 (-7.37, 10.675) -> (-6.72, 10.025) construction
  line L34 (-6.72, 10.675) -> (-7.37, 10.025) construction
  line L35 (3.32, 10.025) -> (2.67, 10.025)
  line L36 (2.67, 10.025) -> (2.67, 17.625)
  line L37 (2.67, 17.625) -> (3.32, 17.625)
  line L38 (3.32, 17.625) -> (3.32, 10.025)
  line L39 (0.81, 10.025) -> (0.16, 10.025)
  line L40 (0.16, 10.025) -> (0.16, 17.625)
  line L41 (0.16, 17.625) -> (0.81, 17.625)
  line L42 (0.81, 17.625) -> (0.81, 10.025)
  line L43 (-1.7, 10.025) -> (-2.35, 10.025)
  line L44 (-2.35, 10.025) -> (-2.35, 17.625)
  line L45 (-2.35, 17.625) -> (-1.7, 17.625)
  line L46 (-1.7, 17.625) -> (-1.7, 10.025)
  line L47 (-4.21, 10.025) -> (-4.86, 10.025)
  line L48 (-4.86, 10.025) -> (-4.86, 17.625)
  line L49 (-4.86, 17.625) -> (-4.21, 17.625)
  line L50 (-4.21, 17.625) -> (-4.21, 10.025)
  line L51 (-6.72, 10.025) -> (-7.37, 10.025)
  line L52 (-7.37, 10.025) -> (-7.37, 17.625)
  line L53 (-7.37, 17.625) -> (-6.72, 17.625)
  line L54 (-6.72, 17.625) -> (-6.72, 10.025)
  point P0 (2.995, 10.35)
  point P1 (0.485, 10.35)
  point P2 (-2.025, 10.35)
  point P3 (-4.535, 10.35)
  point P4 (-7.045, 10.35)
  dimension "d70" = 0.65
  dimension "d71" = 0.65
  dimension "d72" = 0.65
  dimension "d73" = 0.65
  dimension "d74" = 0.65
  dimension "d75" = 0.65
  dimension "d76" = 0.65
  dimension "d77" = 0.65
  dimension "d78" = 0.65
  dimension "d79" = 0.65
  dimension "d80" = 7.6
  dimension "d81" = 7.6
  dimension "d82" = 7.6
  dimension "d83" = 7.6
  dimension "d84" = 7.6
  constraint horizontal L5
  constraint perpendicular L5 L6
  constraint parallel L5 L7
  constraint parallel L6 L8
  constraint coincident L9 P0
  constraint coincident L10 P0
  constraint midpoint L0 P0
  constraint horizontal L11
  constraint perpendicular L11 L12
  constraint parallel L11 L13
  constraint parallel L12 L14
  constraint coincident L15 P1
  constraint coincident L16 P1
  constraint midpoint L1 P1
  constraint horizontal L17
  constraint perpendicular L17 L18
  constraint parallel L17 L19
  constraint parallel L18 L20
  constraint coincident L21 P2
  constraint coincident L22 P2
  constraint midpoint L2 P2
  constraint horizontal L23
  constraint perpendicular L23 L24
  constraint parallel L23 L25
  constraint parallel L24 L26
  constraint coincident L27 P3
  constraint coincident L28 P3
  constraint midpoint L3 P3
  constraint horizontal L29
  constraint perpendicular L29 L30
  constraint parallel L29 L31
  constraint parallel L30 L32
  constraint coincident L33 P4
  constraint coincident L34 P4
  constraint midpoint L4 P4
  constraint horizontal L35
  constraint vertical L36
  constraint horizontal L37
  constraint vertical L38
  constraint horizontal L39
  constraint vertical L40
  constraint horizontal L41
  constraint vertical L42
  constraint horizontal L43
  constraint vertical L44
  constraint horizontal L45
  constraint vertical L46
  constraint horizontal L47
  constraint vertical L48
  constraint horizontal L49
  constraint vertical L50
  constraint horizontal L51
  constraint vertical L52
  constraint horizontal L53
  constraint vertical L54
  measures "d70" distance of L6.end L7.end
  measures "d71" distance of L5.end L6.end
  measures "d72" distance of L12.end L13.end
  measures "d73" distance of L11.end L12.end
  measures "d74" distance of L18.end L19.end
  measures "d75" distance of L17.end L18.end
  measures "d76" distance of L24.end L25.end
  measures "d77" distance of L23.end L24.end
  measures "d78" distance of L30.end L31.end
  measures "d79" distance of L29.end L30.end
  measures "d80" distance of L6.end L37.end
  measures "d81" distance of L12.end L41.end
  measures "d82" distance of L18.end L45.end
  measures "d83" distance of L24.end L49.end
  measures "d84" distance of L30.end L53.end
sketch "PCB Contact Profiles" plane through (7.37, 0, 0) normal (1, 0, 0) x (0, 1, 0)
  line L0 (-17.625, 2.6) -> (-10.025, 2.6)
  line L1 (-10.025, 2.6) -> (-10.025, 4.45)
  line L2 (-10.025, 4.45) -> (-17.625, 4.45)
  line L3 (-17.625, 4.45) -> (-17.625, 2.6)
  line L4 (-10.675, 2.6) -> (-10.675, 4.45)
  line L5 (-10.025, 3.8) -> (-17.625, 3.8)
  dimension "d87" = -0.65
  dimension "d88" = -0.65
sketch "Encoder Shaft" plane through (0, 0, 6.5) normal (0, 0, 1) x (-1, 0, 0)
  line L0 (-7.5, -8.215) -> (-7.25, -8.465) construction
  line L1 (-7.25, -8.465) -> (4.15, -8.465) construction
  line L2 (4.15, -8.465) -> (4.4, -8.215) construction
  line L3 (4.4, -8.215) -> (4.4, 3.185) construction
  line L4 (4.4, 3.185) -> (4.15, 3.435) construction
  line L5 (4.15, 3.435) -> (-7.25, 3.435) construction
  line L6 (-7.25, 3.435) -> (-7.5, 3.185) construction
  line L7 (-7.5, 3.185) -> (-7.5, -8.215) construction
  line L8 (4.4, -2.515) -> (-7.5, -2.515) construction
  circle A0 centre (-1.55, -2.515) radius 3.5
  circle A1 centre (-1.55, -2.515) radius 2
  dimension "d104" = 7
  dimension "d107" = 4
  constraint midpoint L3 L8.start
  constraint midpoint L7 L8.end
  constraint midpoint L8 A0.centre
  constraint concentric A0 A1
  measures "d104" diameter of A0
  measures "d107" diameter of A1
sketch "Shaft II" plane through (0, 0, 14.15) normal (0, 0, 1) x (-1, 0, 0)
  circle A0 centre (-1.55, -2.515) radius 2
  circle A1 centre (-1.55, -2.515) radius 3
  dimension "d110" = 6
  constraint concentric A0 A1
  measures "d110" diameter of A1
sketch "Shaft III" plane through (0, 0, 26.65) normal (0, 0, 1) x (-1, 0, 0)
  circle A0 centre (-1.55, -2.515) radius 3
  line L0 (-1.55, -5.515) -> (-1.55, -1.015) construction
  line L1 (1.0481, -1.015) -> (-4.1481, -1.015)
  dimension "d113" = 4.5
  constraint coincident A0 L0.start
  constraint vertical L0
  constraint perpendicular L0 L1
  constraint midpoint L0.end L1
  constraint coincident A0 L1.end
  measures "d113" distance of L0.start L0.end
ref_plane "WorkPlane1" through (1.55, 0.265, 14) normal (0, 0, 1) x (-1, 0, 0)
sketch "Cap" plane through (1.55, 0.265, 14) normal (0, 0, 1) x (1, 0, 0)
  circle A0 centre (0, 2.25) radius 3 construction
  circle A1 centre (0, 2.25) radius 7.04
  circle A2 centre (0, 2.25) radius 6.49
  dimension "d117" = 14.08
  dimension "d118" = 12.98
  constraint concentric A0 A1
  constraint concentric A1 A2
  measures "d117" diameter of A1
  measures "d118" diameter of A2
extrude "Extrude18" add sketch "Cap" along normal blind 16.6 makes body 1
sketch "Cap II" plane through (0, 0, 30.6) normal (0, 0, 1) x (-1, 0, 0)
  circle A0 centre (-1.55, -2.515) radius 6.49
  circle A1 centre (-1.55, -2.515) radius 7.04
extrude "Extrude19" add sketch "Cap II" against normal blind 13.85 separate body contours A0 makes body 2
combine "Combine7" operation cut target body 2 tool bodies 1 keep tools
combine "Combine8" operation add target body 2 tool bodies 1
sketch "Cap III" plane through (0, 0, 30.6) normal (0, 0, 1) x (-1, 0, 0)
  circle A0 centre (-1.55, -2.515) radius 7.04
  circle A1 centre (-1.55, -2.515) radius 7.405
  circle A2 centre (-1.55, -2.515) radius 7.04
  dimension "d123" = 14.81
  constraint concentric A0 A1
  constraint concentric A1 A2
  measures "d123" diameter of A1
extrude "Extrude20" add sketch "Cap III" against normal blind 12.6 separate body makes body 3
extrude "Extrude21" cut 1 faces at (-0.4232, -4.477, 30.6) along direction (0, 0, -1) blind 1.9 on bodies 3 bodies 3
combine "Combine9" operation add target body 2 tool bodies 3
chamfer "Chamfer7" distance 0.36 angle 45 2 edges at (8.4539, -0.1628, 28.7) (8.4539, -0.1628, 18) on bodies 2